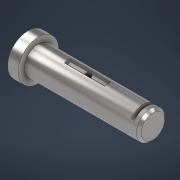
# Autodesk Inventor part: Ось
Saved by Autodesk Inventor 2021 (Build 250183000, 183)
## iProperties
Created: 2022-05-01
Part Number: Ось
Material: Steel, Cast
Document SubType Name: Modeling
Designer: DuctopwH
Density: 7.85 g/cm^3
Appearance: Semi-Polished
Author: DuctopwH
Autodesk Inventor part; units mm, degrees
ref_plane "YZ Plane" through (0, 0, 0) normal (1, 0, 0) x (0, 1, 0)
ref_plane "XZ Plane" through (0, 0, 0) normal (0, 1, 0) x (-1, 0, 0)
ref_plane "XY Plane" through (0, 0, 0) normal (0, 0, 1) x (1, 0, 0)
sketch "Sketch1" plane through (0, 0, 0) normal (0, 0, 1) x (1, 0, 0)
  line L0 (0, 0) -> (-156, 0)
  line L1 (0, 0) -> (0, 14.5)
  line L2 (0, 14.5) -> (-3, 17.5)
  line L3 (-3, 17.5) -> (-142, 17.5)
  line L4 (-142, 17.5) -> (-142, 25)
  line L5 (-142, 25) -> (-155, 25)
  line L6 (-155, 25) -> (-156, 24)
  line L7 (-156, 24) -> (-156, 0)
  dimension "d0" = 35
  dimension "d1" = 3
  dimension "d2" = 45
  dimension "d4" = 14
  dimension "d5" = 156
  dimension "d6" = 50
  dimension "d7" = 45
  dimension "d8" = 1
  constraints: 16 end point, 3 perpendicular, 1 horizontal, 1 parallel, 1 vertical
  measures "d0" diameter of L3 L0
  measures "d1" distance from line of L1 L2.end
  measures "d2" angle of L1 L2
  measures "d4" distance between parallel lines of L7 L4
  measures "d5" distance between parallel lines of L7 L1
  measures "d6" diameter of L5 L0
  measures "d7" angle of L7 L6
  measures "d8" distance from line of L7 L5.end
revolve "Revolution1" add sketch "Sketch1" angle 360 about axis through (0, 0, 0) along (-1, 0, 0)
sketch "Sketch2" plane through (-156, 0, 0) normal (-1, 0, 0) x (0, 0, 1)
  circle A0 centre (0, 0) radius 24 projected
  point P0 (0, 0)
  constraints: 1 coincident
hole "Hole1" at (-156, 0, 0) direction (1, 0, 0) diameter 8 depth 80 tip angle 118
sketch "Sketch3" plane through (0, 0, 0) normal (0, 0, 1) x (1, 0, 0)
  line L0 (-156, -24) -> (-156, 24) projected
  line L1 (-156, 7) -> (-155, 6)
  line L2 (-155, 6) -> (-140, 6)
  line L3 (-140, 6) -> (-140, 4)
  line L4 (-76, 4) -> (-156, 4) projected
  line L5 (-156, 0) -> (-73.5966, 0)
  line L6 (-73.5966, 0) -> (-76, -4) projected
  point P0 (0, 0)
  dimension "d17" = 1
  dimension "d18" = 6
  dimension "d19" = 16
  dimension "d20" = 45
  constraints: 8 end point, 3 point on line, 2 perpendicular, 1 horizontal, 1 midpoint
  measures "d17" horizontal distance of L1.start L1.end
  measures "d18" distance between parallel lines of L5 L2
  measures "d19" distance from line of L0 L2.end
  measures "d20" angle of L0 L1
revolve "Revolution2" cut sketch "Sketch3" angle 360 about axis through (-156, 0, 0) along (1, 0, 0)
sketch "Sketch4" plane through (0, 0, 0) normal (0, 0, 1) x (1, 0, 0)
  line L0 (-142, 17.5) -> (-3, 17.5) projected
  line L1 (-12, 17.5) -> (-12, 9.5)
  line L2 (-12, 9.5) -> (-8, 9.5)
  line L3 (-8, 9.5) -> (-8, 17.5)
  line L4 (0, -14.5) -> (0, 14.5) projected
  point P0 (0, 0)
  dimension "d22" = 4
  dimension "d23" = 12
  dimension "d24" = 8
  constraints: 6 end point, 2 perpendicular, 2 point on line, 1 vertical
  measures "d22" distance between parallel lines of L3 L1
  measures "d23" distance between parallel lines of L4 L1
  measures "d24" distance between parallel lines of L0 L2
extrude "Extrusion1" cut sketch "Sketch4" along normal through all both and the other way through all
sketch "Sketch5" plane through (0, 0, 0) normal (0, 0, 1) x (1, 0, 0)
  line L0 (-76, 4) -> (-140, 4) projected
  line L1 (-81, 4) -> (-81, 17.5)
  line L2 (-142, 17.5) -> (-3, 17.5) projected
  line L3 (-77, 17.5) -> (-77, 4)
  line L4 (-156, -24) -> (-156, 24) projected
  line L5 (-76, -4) -> (-140, -4) projected
  line L6 (-81, 4) -> (-81, -4)
  line L7 (-76, 4) -> (-140, 4) projected
  line L8 (-77, 4) -> (-77, -4)
  line L9 (-81, 0) -> (-77, 0)
  line L10 (-77, 13.5) -> (-81, 13.5)
  point P0 (0, 0)
  dimension "d27" = 4
  dimension "d28" = 75
  dimension "d33" = 4
  constraints: 12 end point, 8 point on line, 5 perpendicular, 2 midpoint
  measures "d27" distance between parallel lines of L3 L1
  measures "d28" distance between parallel lines of L4 L1
  measures "d33" distance between parallel lines of L2 L10
revolve "Revolution3" cut sketch "Sketch5" angle 360 about axis through (-81, 4, 0) along (0, 1, 0) contours L8 L9 L6 L0 | L0 L1 L10 L3 | L10 L1 L2 L3
sketch "Sketch6" plane through (0, 0, 0) normal (0, 0, 1) x (1, 0, 0)
  line L0 (-142, 17.5) -> (-3, 17.5) projected
  line L1 (-106, 17.5) -> (-106, 13.5)
  line L2 (-106, 13.5) -> (-81, 13.5)
  line L3 (-81, 13.5) -> (-56, 13.5)
  line L4 (-56, 13.5) -> (-56, 17.5)
  line L5 (-106, 17.5) -> (-56, 17.5)
  line L6 (-142, 17.5) -> (-3, 17.5) projected
  line L7 (-77, 4) -> (-81, 0) projected
  line L8 (-81, 17.5) -> (-81, 0)
  point P0 (0, 0)
  dimension "d30" = 50
  dimension "d31" = 4
  constraints: 12 end point, 4 point on line, 3 perpendicular, 1 collinear, 1 midpoint, 1 vertical
  measures "d30" distance between parallel lines of L4 L1
  measures "d31" distance between parallel lines of L0 L2
revolve "Revolution4" cut sketch "Sketch6" angle 360 about axis through (-142, 17.5, 0) along (1, 0, 0)
body "Solid1"
